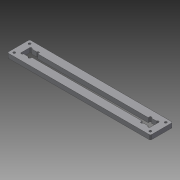
# Autodesk Inventor part: Arrow_Arm_Template
Saved by Autodesk Inventor 2014 (Build 180170000, 170)
## iProperties
Created: 2014-10-25
Part Number: Arrow_Arm_Template
Material: Generic
Document SubType Name: Modeling
Designer: ThatOtherGuy
Density: 1 g/cm^3
Appearance: Default
Author: ThatOtherGuy
Autodesk Inventor part; units mm, degrees
ref_plane "YZ Plane" through (0, 0, 0) normal (1, 0, 0) x (0, 1, 0)
ref_plane "XZ Plane" through (0, 0, 0) normal (0, 1, 0) x (-1, 0, 0)
ref_plane "XY Plane" through (0, 0, 0) normal (0, 0, 1) x (1, 0, 0)
sketch "Sketch1" plane through (0, 0, 0) normal (0, 0, 1) x (1, 0, 0)
  line L0 (0, 0) -> (102.5, 0)
  line L1 (0, 0) -> (0, 16)
  line L2 (0, 4.2898) -> (79, 4.2898)
  line L3 (79, 4.2898) -> (79, 6)
  line L4 (79, 6) -> (92.5, 6)
  line L5 (92.5, 6) -> (92.5, 0)
  line L6 (0, 16) -> (102.5, 16)
  line L7 (102.5, 16) -> (102.5, 0)
  circle A0 centre (97.5, 11) radius 1.5875
  dimension "d0" = 13.5
  dimension "d1" = 12
  dimension "d2" = 8.5796
  dimension "d3" = 185
  dimension "d4" = 10
  dimension "d5" = 10
  dimension "d6" = 3.175
  dimension "d7" = 5
  dimension "d8" = 5
  constraints: 16 end point, 5 perpendicular, 2 parallel, 2 point on line, 1 centre point, 1 horizontal, 1 vertical
  measures "d0" distance of L3.end L4.end
  measures "d1" diameter of L4 L0
  measures "d2" diameter of L2 L0
  measures "d3" diameter of L5 L1
  measures "d4" distance between parallel lines of L7 L5
  measures "d5" distance between parallel lines of L6 L4
  measures "d6" diameter of A0
  measures "d7" distance from line of L6 A0.centre
  measures "d8" distance from line of L7 A0.centre
extrude "Extrusion1" add sketch "Sketch1" along normal blind 6.35 contours L5 L4 L3 L2 L1 L6 L7 L0
sketch "Sketch2" plane through (0, 0, 6.35) normal (0, 0, 1) x (1, 0, 0)
  line L0 (79, 4.2898) -> (79, 6) projected
  line L1 (79, 6) -> (92.5, 6) projected
  line L2 (92.5, 6) -> (92.5, 0) projected
  arc A0 (82.175, 6) -> (79, 6) centre (80.5875, 6) ccw
  arc A1 (92.5, 6) -> (89.325, 6) centre (90.9125, 6) ccw
  point P0 (0, 0)
  dimension "d12" = 1.5875
  constraints: 4 point on circle, 2 centre point, 2 point on line, 2 tangent, 1 equal radius
  measures "d12" radius of A0
extrude "Extrusion2" cut sketch "Sketch2" against normal up to next
fillet "Fillet1" radius 2 1 edges at (102.5, 16, 3.175)
mirror "Mirror1" about plane through (92.5, 0, 0) normal (0, -1, 0) of "Extrusion1", "Fillet1", "Extrusion2"
mirror "Mirror2" about plane through (0, -16, 0) normal (-1, 0, 0) of "Extrusion1", "Fillet1", "Mirror1", "Extrusion2"
body "Solid1"
